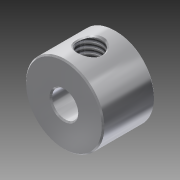
# Autodesk Inventor part: 08-0003
Saved by Autodesk Inventor 2015 SP1 (Build 190203100, 203)
## iProperties
Category: Axle Collar Service Pack
Company: Autodesk Inc.
Created: 2014-11-30
Part Number: 08-0003
Material: Aluminum 6061
Document SubType Name: Modeling
Designer: Matrix
Density: 2.7 g/cm^3
Appearance: Aluminum - Polished
Catalog Web Link: http://matrixrobotics.com/
Vendor: Matrix
Author: Autodesk Inc.
Autodesk Inventor part; units mm, degrees
note: some values were not read from the file. Chosen so that the rebuilt part matches the saved one: direction of "Hole2".
ref_plane "YZ Plane" through (0, 0, 0) normal (1, 0, 0) x (0, 1, 0)
ref_plane "XZ Plane" through (0, 0, 0) normal (0, 1, 0) x (-1, 0, 0)
sketch "Sketch1" plane through (0, 0, 0) normal (0, 1, 0) x (-1, 0, 0)
  circle A0 centre (0, 0) radius 6
  dimension "d0" = 12
  constraints: 1 centre point, 1 coincident
  measures "d0" diameter of A0
extrude "Extrusion1" add sketch "Sketch1" against normal blind 8
chamfer "Chamfer1" distance 0.2 angle 45 2 edges at (6, -8, 0) (6, 0, 0)
sketch "Sketch2" plane through (0, -8, 0) normal (0, -1, 0) x (1, 0, 0)
  point P0 (0, 0)
hole "Hole1" at (0, -8, 0) direction (0, 1, 0) diameter 4 end through all
chamfer "Chamfer2" distance 0.2 angle 45 2 edges at (0, -8, 2) (0, 0, 2)
ref_plane "Work Plane1" through (0, 0, 6) normal (0, 0, 1) x (1, 0, 0)
sketch "Sketch3" plane through (0, 0, 6) normal (0, 0, 1) x (1, 0, 0)
  line L0 (-6, -0.2) -> (-6, -7.8) projected
  line L1 (-5.8, 0) -> (5.8, 0) projected
  point P0 (0, 0)
  point P1 (0, -4)
  point P2 (-6, -4)
  constraints: 1 horizontal alignment, 1 midpoint, 1 vertical alignment
hole "Hole2" at (0, -4, 6) direction (0, 0, -1) diameter 3.688 end up to surface thread size "M4.5x0.75" class "6H" standard "ANSI Metric M Profile"
chamfer "Chamfer3" distance 0.2 angle 45 2 edges at (1.8366, -3.8348, 5.712) (-1.844, -4.0029, 5.7096)
body "Solid1"
